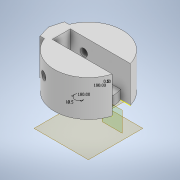
# Autodesk Inventor part: handle_base
Saved by Autodesk Inventor 2021 (Build 250183000, 183)
## iProperties
Created: 2021-03-06
Part Number: handle_base
Material: Generic
Document SubType Name: Modeling
Designer: ben
Density: 1 g/cm^3
Appearance: Default
Mass: 226.368 g
Surface Area: 425.082 cm^2
Volume: 226.368 cm^3
Author: ben
Autodesk Inventor part; units mm, degrees
ref_plane "YZ Plane" through (0, 0, 0) normal (1, 0, 0) x (0, 1, 0)
ref_plane "XZ Plane" through (0, 0, 0) normal (0, 1, 0) x (-1, 0, 0)
ref_plane "XY Plane" through (0, 0, 0) normal (0, 0, 1) x (1, 0, 0)
ref_plane "Work Plane1" through (-35, 22.5, -35) normal (0, 0, 1) x (1, 0, 0)
sketch "Sketch1" plane through (-35, 22.5, -35) normal (0, 0, 1) x (1, 0, 0)
  circle A0 centre (35, -42) radius 27.25
  circle A1 centre (35, -42) radius 6
  dimension "d0" = 54.5
  dimension "d24" = 12
  constraints: 2 centre point, 1 coincident, 1 other
  measures "d0" diameter of A0
  measures "d24" diameter of A1
ref_plane "Work Plane2" through (0, -19.5, 0) normal (0, 0, 1) x (1, 0, 0)
sketch "Sketch2" plane through (0, -19.5, 0) normal (0, 0, 1) x (1, 0, 0)
  arc A0 (-36.1421, -10) -> (-36.1421, 10) centre (0, 0) ccw
  line L0 (29.9857, -10) -> (-36.1421, -10)
  line L1 (-36.1421, 10) -> (29.9857, 10)
  line L2 (29.9857, 10) -> (29.9857, -10)
  line L3 (34.9857, -13.5) -> (39.9857, -13.5)
  line L4 (39.9857, -13.5) -> (39.9857, 13.5)
  line L5 (39.9857, 13.5) -> (34.9857, 13.5)
  line L6 (34.9857, 13.5) -> (34.9857, -13.5)
  line L7 (39.9857, -13.5) -> (43.6938, 0)
  line L8 (43.6938, 0) -> (39.9857, 13.5)
  point P0 (0, 19.5)
  point P1 (37.5, 0)
  point P2 (36.1421, 10)
  point P3 (36.1421, -10)
  dimension "d3" = 75
  dimension "d40" = 5
  dimension "d41" = 27
  dimension "d44" = 14
  dimension "d110" = 5
  constraints: 18 end point, 4 horizontal, 4 point on circle, 3 parallel, 1 centre point, 1 perpendicular, 1 vertical, 1 other
  measures "d3" diameter of A0
  measures "d40" distance of L3.start L3.end
  measures "d41" distance of L5.end L3.start
  measures "d44" distance of L3.end L7.end
  measures "d110" distance between parallel lines of L2 L6
extrude "Extrusion2" add sketch "Sketch2" along normal blind 40
ref_plane "Work Plane3" through (-36.1421, -9.5, 0) normal (0, -1, 0) x (1, 0, 0)
sketch "Sketch4" plane through (-36.1421, -9.5, 0) normal (0, -1, 0) x (1, 0, 0)
  line L0 (0, 0) -> (10.5247, 0) projected
  line L1 (0, 0) -> (66.1278, 0) projected
  line L2 (66.1278, 0) -> (66.1278, 40) projected
  line L3 (0, 40) -> (66.1278, 40) projected
  line L4 (0, 0) -> (0, 40) projected
  line L5 (0, 10) -> (66.1278, 10)
  line L6 (66.1278, 0) -> (66.1278, 40) projected
  point P0 (36.1421, 0)
  point P1 (51.1278, 25)
  dimension "d99" = 15
  dimension "d100" = 10
  dimension "d101" = 15
  constraints: 2 end point, 2 point on line, 1 horizontal
  measures "d99" distance from line of L2 point (51.128, 25)
  measures "d100" distance between parallel lines of L1 L5
  measures "d101" distance from line of L5 point (51.128, 25)
hole "Hole2" at (14.9857, -9.5, 25) direction (0, 1, 0) diameter 8.1 end through all both
extrude "Extrusion3" add sketch "Sketch1" along normal blind 35 and the other way blind 10
sketch "Sketch8" plane through (0, -19.5, -45) normal (0, 0, -1) x (-1, 0, 0)
  circle A0 centre (0, 0) radius 6 projected
  circle A1 centre (0, 0) radius 6 projected
  line L0 (7.1547, 0) -> (5.4226, -1)
  line L1 (5.4226, -1) -> (5.4226, 1)
  line L2 (5.4226, 1) -> (7.1547, 0)
  line L3 (5.0591, 5.0591) -> (4.5415, 3.1273)
  line L4 (4.5415, 3.1273) -> (3.1273, 4.5415)
  line L5 (3.1273, 4.5415) -> (5.0591, 5.0591)
  line L6 (0, 7.1547) -> (1, 5.4226)
  line L7 (1, 5.4226) -> (-1, 5.4226)
  line L8 (-1, 5.4226) -> (0, 7.1547)
  line L9 (-5.0591, 5.0591) -> (-3.1273, 4.5415)
  line L10 (-3.1273, 4.5415) -> (-4.5415, 3.1273)
  line L11 (-4.5415, 3.1273) -> (-5.0591, 5.0591)
  line L12 (-7.1547, 0) -> (-5.4226, 1)
  line L13 (-5.4226, 1) -> (-5.4226, -1)
  line L14 (-5.4226, -1) -> (-7.1547, 0)
  line L15 (-5.0591, -5.0591) -> (-4.5415, -3.1273)
  line L16 (-4.5415, -3.1273) -> (-3.1273, -4.5415)
  line L17 (-3.1273, -4.5415) -> (-5.0591, -5.0591)
  line L18 (0, -7.1547) -> (-1, -5.4226)
  line L19 (-1, -5.4226) -> (1, -5.4226)
  line L20 (1, -5.4226) -> (0, -7.1547)
  line L21 (5.0591, -5.0591) -> (3.1273, -4.5415)
  line L22 (3.1273, -4.5415) -> (4.5415, -3.1273)
  line L23 (4.5415, -3.1273) -> (5.0591, -5.0591)
  circle A2 centre (0, 0) radius 27.25 projected
  circle A3 centre (0, 0) radius 29.25
  line L24 (5.3226, -1.1732) -> (7.3547, 0)
  line L25 (7.3547, 0) -> (5.3226, 1.1732)
  line L26 (5.3226, 1.1732) -> (5.3226, -1.1732)
  line L27 (5.2006, 5.2006) -> (2.9341, 4.5933)
  line L28 (4.5933, 2.9341) -> (5.2006, 5.2006)
  line L29 (2.9341, 4.5933) -> (4.5933, 2.9341)
  line L30 (0, 7.3547) -> (-1.1732, 5.3226)
  line L31 (1.1732, 5.3226) -> (0, 7.3547)
  line L32 (-1.1732, 5.3226) -> (1.1732, 5.3226)
  line L33 (-5.2006, 5.2006) -> (-4.5933, 2.9341)
  line L34 (-2.9341, 4.5933) -> (-5.2006, 5.2006)
  line L35 (-4.5933, 2.9341) -> (-2.9341, 4.5933)
  line L36 (-7.3547, 0) -> (-5.3226, -1.1732)
  line L37 (-5.3226, 1.1732) -> (-7.3547, 0)
  line L38 (-5.3226, -1.1732) -> (-5.3226, 1.1732)
  line L39 (-5.2006, -5.2006) -> (-2.9341, -4.5933)
  line L40 (-4.5933, -2.9341) -> (-5.2006, -5.2006)
  line L41 (-2.9341, -4.5933) -> (-4.5933, -2.9341)
  line L42 (0, -7.3547) -> (1.1732, -5.3226)
  line L43 (-1.1732, -5.3226) -> (0, -7.3547)
  line L44 (1.1732, -5.3226) -> (-1.1732, -5.3226)
  line L45 (5.2006, -5.2006) -> (4.5933, -2.9341)
  line L46 (2.9341, -4.5933) -> (5.2006, -5.2006)
  line L47 (4.5933, -2.9341) -> (2.9341, -4.5933)
  point P0 (0, 19.5)
  point P1 (-6, 0)
  point P2 (6, 0)
  point P3 (4.2426, 4.2426)
  point P4 (0, 6)
  point P5 (-4.2426, 4.2426)
  point P6 (-6, 0)
  point P7 (-4.2426, -4.2426)
  point P8 (0, -6)
  point P9 (4.2426, -4.2426)
  point P10 (4.7022, -3.7269)
  point P11 (3.7269, -4.7022)
  point P12 (0.6896, -5.9602)
  point P13 (-0.6896, -5.9602)
  point P14 (-3.7269, -4.7022)
  point P15 (-4.7022, -3.7269)
  point P16 (-5.9602, -0.6896)
  point P17 (-5.9602, 0.6896)
  point P18 (-4.7022, 3.7269)
  point P19 (-3.7269, 4.7022)
  point P20 (-0.6896, 5.9602)
  point P21 (0.6896, 5.9602)
  point P22 (3.7269, 4.7022)
  point P23 (4.7022, 3.7269)
  point P24 (5.9602, 0.6896)
  point P25 (5.9602, -0.6896)
  point P26 (3.6277, -4.7791)
  point P27 (0.8142, -5.9445)
  point P28 (-0.8142, -5.9445)
  point P29 (-3.6277, -4.7791)
  point P30 (-4.7791, -3.6277)
  point P31 (-5.9445, -0.8142)
  point P32 (-5.9445, 0.8142)
  point P33 (-4.7791, 3.6277)
  point P34 (-3.6277, 4.7791)
  point P35 (-0.8142, 5.9445)
  point P36 (0.8142, 5.9445)
  point P37 (3.6277, 4.7791)
  point P38 (4.7791, 3.6277)
  point P39 (5.9445, 0.8142)
  point P40 (5.9445, -0.8142)
  point P41 (4.7791, -3.6277)
  dimension "d102" = 2
  dimension "d105" = 360
  dimension "d107" = 2
  dimension "d115" = 0.1
  dimension "d118" = 360
  constraints: 96 end point, 2 point on circle, 1 centre point, 1 coincident, 116 other
  measures "d102" distance of L0.end L1.end
  measures "d107" radial gap between concentric circles of A2 A3
  measures "d115" distance between parallel lines of L0 L24
ref_plane "Work Plane4" through (-35, 22.5, 0) normal (0, 0, 1) x (1, 0, 0)
split body "Split1" result two bodies by plane through (-35, 22.5, 0) normal (0, 0, 1) first body at (5.2266, -56.129, 21.6332)
sketch "top-bottom notch" plane through (0, -19.5, 0) normal (0, 0, 1) x (1, 0, 0)
  arc A0 (-10, -10) -> (10, -10) centre (0, -10) ccw
  line L0 (0, -10) -> (-10, -10) construction
  line L1 (0, -10) -> (10, -10) construction
  line L2 (29.9857, -10) -> (-36.1421, -10) projected
  line L3 (-36.1421, 10) -> (29.9857, 10) projected
  arc A1 (10, 10) -> (-10, 10) centre (0, 10) ccw
  line L4 (0, 10) -> (-10, 10) construction
  line L5 (0, 10) -> (10, 10) construction
  arc A2 (-9.4868, -10.5) -> (9.4868, -10.5) centre (0, -10) ccw
  line L6 (-9.4868, -10.5) -> (0, -10.5)
  line L7 (0, -10.5) -> (9.4868, -10.5)
  arc A3 (9.4868, 10.5) -> (-9.4868, 10.5) centre (0, 10) ccw
  line L8 (9.4868, 10.5) -> (0, 10.5)
  line L9 (0, 10.5) -> (-9.4868, 10.5)
  point P0 (-10, -10)
  point P1 (-10, 10)
  dimension "d87" = 10
  dimension "d88" = 180
  dimension "d89" = 10
  dimension "d90" = 180
  dimension "d91" = 0.5
  dimension "d92" = 0.5
  constraints: 16 end point, 8 point on circle, 4 centre point, 3 point on line, 4 other
  measures "d87" radius of A0
  measures "d88" angle of L1 L0
  measures "d89" radius of A1
  measures "d90" angle of L4 L5
  measures "d91" radial gap between concentric circles of A0 A2
  measures "d92" radial gap between concentric circles of A1 A3
extrude "Extrusion10" add sketch "top-bottom notch" against normal blind 5 contours L6 L7 A2 | L8 L9 A3 bodies 2
extrude "Extrusion11" cut sketch "top-bottom notch" against normal blind 7 contours L2 A0 | A1 L3 | L6 L7 A2 | L8 L9 A3 bodies 3
sketch "Sketch15" plane through (0, -19.5, 0) normal (0, 0, -1) x (-1, 0, 0)
  line L0 (10, -10) -> (-10, -10) projected
  arc A0 (-10, -10) -> (10, -10) centre (0, -10) ccw projected
  arc A1 (10, 10) -> (-10, 10) centre (0, 10) ccw projected
  line L1 (-10, 10) -> (10, 10) projected
  circle A2 centre (0, 0) radius 6 projected
  circle A3 centre (0, 0) radius 27.25 projected
  line L2 (-29.9857, -10) -> (36.1421, -10) projected
  line L3 (36.1421, 10) -> (-29.9857, 10) projected
  point P0 (0, 19.5)
  point P1 (-25.3488, 10)
  point P2 (-25.3488, -10)
  point P3 (25.3488, -10)
  point P4 (25.3488, 10)
extrude "Extrusion12" add sketch "Sketch15" against normal blind 10 contours L0 L2 A3 L3 L1 bodies 2
extrude "Extrusion13" add sketch "Sketch8" along normal blind 2 contours A2 | A3 bodies 3
ref_plane "Work Plane5" through (0, -19.5, -35) normal (0, 0, 1) x (1, 0, 0)
sketch "Sketch16" plane through (0, -19.5, -35) normal (0, 0, 1) x (1, 0, 0)
  circle A0 centre (0, 0) radius 6 projected
  circle A1 centre (0, 0) radius 4
  point P0 (0, 19.5)
  dimension "d112" = 8
  constraints: 1 centre point, 1 coincident
  measures "d112" diameter of A1
extrude "Extrusion14" add sketch "Sketch16" against normal blind 5 bodies 3
